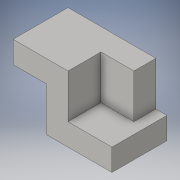
# Autodesk Inventor part: Figure 7_27_8
Saved by Autodesk Inventor 2016 (Build 200138000, 138)
## iProperties
Created: 2016-07-18
Part Number: Figure 7_27_8
Material: Generic
Document SubType Name: Modeling
Designer: cfkguest
Density: 1 g/cm^3
Appearance: Default
Author: cfkguest
Autodesk Inventor part; units mm, degrees
ref_plane "YZ Plane" through (0, 0, 0) normal (1, 0, 0) x (0, 1, 0)
ref_plane "XZ Plane" through (0, 0, 0) normal (0, 1, 0) x (-1, 0, 0)
ref_plane "XY Plane" through (0, 0, 0) normal (0, 0, 1) x (1, 0, 0)
sketch "Sketch1" plane through (0, 0, 0) normal (0, 0, 1) x (1, 0, 0)
  line L0 (-35.6004, 16.8538) -> (21.5496, 16.8538)
  line L1 (21.5496, 16.8538) -> (21.5496, -21.2462)
  line L2 (21.5496, -21.2462) -> (-35.6004, -21.2462)
  line L3 (-35.6004, -21.2462) -> (-35.6004, 16.8538)
  point P0 (0, 0)
  dimension "d0" = 57.15
  dimension "d1" = 38.1
  constraints: 8 end point, 2 parallel, 1 horizontal, 1 perpendicular
  measures "d0" distance of L0.start L0.end
  measures "d1" distance of L0.end L1.end
extrude "Extrusion1" add sketch "Sketch1" along normal blind 31.75
sketch "Sketch2" plane through (21.5496, -21.2462, 0) normal (1, 0, 0) x (0, 0, -1)
  line L0 (0, 0) -> (0, 38.1) projected
  line L1 (0, 38.1) -> (-12.7, 38.1)
  line L2 (-12.7, 38.1) -> (-12.7, 12.7)
  line L3 (-12.7, 12.7) -> (0, 12.7)
  line L4 (0, 12.7) -> (0, 38.1)
  point P0 (0, 21.2462)
  dimension "d4" = 25.4
  dimension "d5" = 12.7
  constraints: 8 end point, 2 parallel, 1 horizontal, 1 perpendicular
  measures "d4" distance of L1.end L2.end
  measures "d5" distance of L2.end L3.end
extrude "Extrusion2" cut sketch "Sketch2" against normal blind 6.35
sketch "Sketch3" plane through (-35.6004, 16.8538, 31.75) normal (0, 1, 0) x (1, 0, 0)
  line L0 (57.15, 31.75) -> (57.15, 0) projected
  line L1 (57.15, 0) -> (31.75, 0)
  line L2 (31.75, 0) -> (31.75, 19.05)
  line L3 (31.75, 19.05) -> (57.15, 19.05)
  line L4 (57.15, 19.05) -> (57.15, 0)
  point P0 (35.6004, 31.75)
  dimension "d8" = 19.05
  dimension "d9" = 25.4
  constraints: 8 end point, 2 parallel, 1 horizontal, 1 perpendicular
  measures "d8" distance of L1.end L2.end
  measures "d9" distance of L2.end L3.end
extrude "Extrusion3" cut sketch "Sketch3" against normal blind 25.4
sketch "Sketch4" plane through (0, 0, 31.75) normal (0, 0, 1) x (1, 0, 0)
  line L0 (-35.6004, -21.2462) -> (-16.5504, -21.2462)
  line L1 (-16.5504, -21.2462) -> (-16.5504, 4.1538)
  line L2 (-16.5504, 4.1538) -> (-35.6004, 4.1538)
  line L3 (-35.6004, 4.1538) -> (-35.6004, -21.2462)
  point P0 (0, 0)
  dimension "d12" = 19.05
  dimension "d13" = 25.4
  constraints: 8 end point, 2 parallel, 1 horizontal, 1 perpendicular
  measures "d12" distance of L1.end L2.end
  measures "d13" distance of L0.end L1.end
extrude "Extrusion4" cut sketch "Sketch4" against normal blind 50.8
body "Solid1"
